Autodesk Fusion 360 part; units mm, degrees
(part 3 of 3)
  spline S752 degree 3 poles (35.1137, 3.9939) (35.046, 4.0714) (34.9934, 4.0943) (34.9088, 4.0943) knots 0 0 0 0 1 1 1 1
  spline S753 degree 3 poles (37.0883, 3.2718) (37.0935, 3.2826) (37.1011, 3.3047) (37.1069, 3.3369) knots 0 0 0 0 0.456304 0.456304 0.456304 0.456304
  spline S754 degree 3 poles (37.1069, 3.3369) (37.0284, 3.3202) (36.9414, 3.3052) (36.8456, 3.2915) knots 0.585455 0.585455 0.585455 0.585455 0.999639 0.999639 0.999639 0.999639
  spline S755 degree 3 poles (36.8456, 3.2915) (36.7271, 3.2744) (36.6453, 3.2517) (36.629, 3.2446) knots 0 0 0 0 1 1 1 1
  spline S756 degree 3 poles (36.629, 3.2446) (36.6076, 3.2353) (36.6025, 3.2294) (36.5959, 3.2194) knots 0.000036 0.000036 0.000036 0.000036 1 1 1 1
  spline S757 degree 3 poles (36.5959, 3.2194) (36.5878, 3.2068) (36.5856, 3.2004) (36.5856, 3.1825) knots 0.000113 0.000113 0.000113 0.000113 1 1 1 1
  spline S758 degree 3 poles (36.5856, 3.1825) (36.5856, 3.1511) (36.586, 3.1497) (36.6107, 3.1279) knots 0 0 0 0 1 1 1 1
  spline S759 degree 3 poles (36.6107, 3.1279) (36.6249, 3.1155) (36.6616, 3.096) (36.7505, 3.096) knots 0.000045 0.000045 0.000045 0.000045 1 1 1 1
  spline S760 degree 3 poles (36.7505, 3.096) (36.8396, 3.096) (36.9078, 3.1141) (36.968, 3.1479) knots 0 0 0 0 1 1 1 1
  spline S761 degree 3 poles (36.968, 3.1479) (37.0284, 3.1818) (37.0627, 3.2189) (37.0883, 3.2718) knots 0.000007 0.000007 0.000007 0.000007 0.994861 0.994861 0.994861 0.994861
  spline S762 degree 3 poles (37.8884, 11.0482) (37.867, 11.0389) (37.8618, 11.0329) (37.8553, 11.0229) knots 0.000005 0.000005 0.000005 0.000005 1 1 1 1
  spline S763 degree 3 poles (37.8553, 11.0229) (37.8471, 11.0103) (37.845, 11.004) (37.845, 10.986) knots 0 0 0 0 1 1 1 1
  spline S764 degree 3 poles (37.845, 10.986) (37.845, 10.9546) (37.8453, 10.9533) (37.8701, 10.9315) knots 0 0 0 0 1 1 1 1
  spline S765 degree 3 poles (37.8701, 10.9315) (37.8842, 10.919) (37.921, 10.8995) (38.0099, 10.8995) knots 0 0 0 0 1 1 1 1
  spline S766 degree 3 poles (38.0099, 10.8995) (38.099, 10.8995) (38.1672, 10.9177) (38.2274, 10.9515) knots 0 0 0 0 1 1 1 1
  spline S767 degree 3 poles (38.2274, 10.9515) (38.2878, 10.9854) (38.3221, 11.0224) (38.3477, 11.0753) knots 0 0 0 0 0.994864 0.994864 0.994864 0.994864
  spline S768 degree 3 poles (38.3477, 11.0753) (38.3528, 11.0862) (38.3605, 11.1082) (38.3663, 11.1404) knots 0 0 0 0 0.4563 0.4563 0.4563 0.4563
  spline S769 degree 3 poles (38.3663, 11.1404) (38.2878, 11.1238) (38.2008, 11.1087) (38.1049, 11.095) knots 0.585457 0.585457 0.585457 0.585457 0.999641 0.999641 0.999641 0.999641
  spline S770 degree 3 poles (38.1049, 11.095) (37.9865, 11.078) (37.9046, 11.0552) (37.8884, 11.0482) knots 0 0 0 0 1 1 1 1
  spline S771 degree 3 poles (41.9828, 11.4158) (41.9828, 11.6094) (41.9395, 11.7253) (41.8802, 11.7925) knots 0 0 0 0 1 1 1 1
  spline S772 degree 3 poles (41.8802, 11.7925) (41.8109, 11.8711) (41.7511, 11.8979) (41.6507, 11.8979) knots 0 0 0 0 1 1 1 1
  spline S773 degree 3 poles (41.6507, 11.8979) (41.5471, 11.8979) (41.4868, 11.8706) (41.4188, 11.7934) knots 0 0 0 0 1 1 1 1
  spline S774 degree 3 poles (41.4188, 11.7934) (41.3618, 11.7287) (41.317, 11.6084) (41.317, 11.4055) knots 0.000006 0.000006 0.000006 0.000006 1 1 1 1
  spline S775 degree 3 poles (41.317, 11.4055) (41.317, 11.2027) (41.3617, 11.0819) (41.4191, 11.0164) knots 0 0 0 0 1 1 1 1
  spline S776 degree 3 poles (41.4191, 11.0164) (41.4873, 10.9387) (41.5474, 10.9115) (41.6507, 10.9115) knots 0.000005 0.000005 0.000005 0.000005 1 1 1 1
  spline S777 degree 3 poles (41.6507, 10.9115) (41.7523, 10.9115) (41.8118, 10.9384) (41.8803, 11.0169) knots 0 0 0 0 1 1 1 1
  spline S778 degree 3 poles (41.8803, 11.0169) (41.937, 11.0819) (41.9828, 11.2065) (41.9828, 11.4158) knots 0.000006 0.000006 0.000006 0.000006 1 1 1 1
  spline S779 degree 3 poles (39.2584, 7.9101) (39.1924, 7.9899) (39.1461, 8.0098) (39.0723, 8.0098) knots 0.000011 0.000011 0.000011 0.000011 1 1 1 1
  spline S780 degree 3 poles (39.0723, 8.0098) (39.0039, 8.0098) (38.9533, 7.9887) (38.8797, 7.8993) knots 0 0 0 0 1 1 1 1
  spline S781 degree 3 poles (38.8797, 7.8993) (38.8187, 7.8253) (38.7744, 7.6978) (38.7744, 7.4935) knots 0.00001 0.00001 0.00001 0.00001 1 1 1 1
  spline S782 degree 3 poles (38.7744, 7.4935) (38.7744, 7.2875) (38.8186, 7.165) (38.8685, 7.1061) knots 0 0 0 0 1 1 1 1
  spline S783 degree 3 poles (38.8685, 7.1061) (38.9327, 7.0303) (38.9799, 7.0097) (39.0587, 7.0097) knots 0.000011 0.000011 0.000011 0.000011 1 1 1 1
  spline S784 degree 3 poles (39.0587, 7.0097) (39.1387, 7.0097) (39.1886, 7.0315) (39.2561, 7.1116) knots 0 0 0 0 1 1 1 1
  spline S785 degree 3 poles (39.2561, 7.1116) (39.3089, 7.1743) (39.3549, 7.3037) (39.3549, 7.5191) knots 0 0 0 0 1 1 1 1
  spline S786 degree 3 poles (39.3549, 7.5191) (39.3549, 7.7225) (39.3114, 7.846) (39.2584, 7.9101) knots 0 0 0 0 1 1 1 1
  spline S787 degree 3 poles (43.6795, 7.9136) (43.6679, 7.9022) (43.6578, 7.8905) (43.6483, 7.8777) knots 0 0 0 0 0.197473 0.197473 0.197473 0.197473
  line L387 (43.6483, 7.8777) -> (44.1325, 7.8777)
  spline S788 degree 3 poles (44.1325, 7.8777) (44.1293, 7.8826) (44.1262, 7.8868) (44.1231, 7.8906) knots 0.866058 0.866058 0.866058 0.866058 0.982774 0.982774 0.982774 0.982774
  spline S789 degree 3 poles (44.1231, 7.8906) (44.1225, 7.8914) (44.1218, 7.8922) (44.1211, 7.893) (44.0566, 7.9711) (44.0001, 7.9978) (43.895, 7.9978) knots -0.006904 -0.006904 -0.006904 -0.006904 0 0 0 1 1 1 1
  spline S790 degree 3 poles (43.895, 7.9978) (43.7986, 7.9978) (43.7407, 7.9737) (43.6795, 7.9136) knots 0 0 0 0 1 1 1 1
  spline S791 degree 3 poles (40.3914, 4.0943) (40.2878, 4.0943) (40.2275, 4.0671) (40.1594, 3.9899) knots 0 0 0 0 1 1 1 1
  spline S792 degree 3 poles (40.1594, 3.9899) (40.1024, 3.9252) (40.0576, 3.8048) (40.0576, 3.602) knots 0.000005 0.000005 0.000005 0.000005 1 1 1 1
  spline S793 degree 3 poles (40.0576, 3.602) (40.0576, 3.3991) (40.1024, 3.2783) (40.1598, 3.2129) knots 0 0 0 0 1 1 1 1
  spline S794 degree 3 poles (40.1598, 3.2129) (40.2279, 3.1352) (40.288, 3.1079) (40.3914, 3.1079) knots 0.000003 0.000003 0.000003 0.000003 1 1 1 1
  spline S795 degree 3 poles (40.3914, 3.1079) (40.493, 3.1079) (40.5525, 3.1349) (40.621, 3.2133) knots 0 0 0 0 1 1 1 1
  spline S796 degree 3 poles (40.621, 3.2133) (40.6777, 3.2783) (40.7234, 3.403) (40.7234, 3.6122) knots 0.000006 0.000006 0.000006 0.000006 1 1 1 1
  spline S797 degree 3 poles (40.7234, 3.6122) (40.7234, 3.8059) (40.6801, 3.9217) (40.6208, 3.989) knots 0 0 0 0 1 1 1 1
  spline S798 degree 3 poles (40.6208, 3.989) (40.5515, 4.0675) (40.4917, 4.0943) (40.3914, 4.0943) knots 0 0 0 0 1 1 1 1
  spline S799 degree 3 poles (45.0503, 4.0943) (44.9467, 4.0943) (44.8864, 4.0671) (44.8184, 3.9899) knots 0 0 0 0 1 1 1 1
  spline S800 degree 3 poles (44.8184, 3.9899) (44.7613, 3.9252) (44.7165, 3.8048) (44.7165, 3.602) knots 0.000005 0.000005 0.000005 0.000005 1 1 1 1
  spline S801 degree 3 poles (44.7165, 3.602) (44.7165, 3.3991) (44.7613, 3.2783) (44.8187, 3.2129) knots 0 0 0 0 1 1 1 1
  spline S802 degree 3 poles (44.8187, 3.2129) (44.8868, 3.1352) (44.947, 3.1079) (45.0503, 3.1079) knots 0.000003 0.000003 0.000003 0.000003 1 1 1 1
  spline S803 degree 3 poles (45.0503, 3.1079) (45.1519, 3.1079) (45.2114, 3.1349) (45.2799, 3.2133) knots 0 0 0 0 1 1 1 1
  spline S804 degree 3 poles (45.2799, 3.2133) (45.3366, 3.2783) (45.3824, 3.403) (45.3824, 3.6122) knots 0.000006 0.000006 0.000006 0.000006 1 1 1 1
  spline S805 degree 3 poles (45.3824, 3.6122) (45.3824, 3.8059) (45.339, 3.9217) (45.2797, 3.989) knots 0 0 0 0 1 1 1 1
  spline S806 degree 3 poles (45.2797, 3.989) (45.2105, 4.0675) (45.1506, 4.0943) (45.0503, 4.0943) knots 0 0 0 0 1 1 1 1
  dimension "d2" = 60
  dimension "d3" = 1
  dimension "d5" = 35
  dimension "d7" = 5
  dimension "d18" = -0.2
  dimension "d19" = -0.2
  dimension "d20" = -0.2
  dimension "d21" = -0.2
  dimension "d22" = -0.2
  dimension "d23" = -0.2
  dimension "d24" = -0.2
  dimension "d25" = -0.2
  dimension "d26" = -0.2
  dimension "d27" = -0.2
  dimension "d28" = -0.2
  dimension "d29" = -0.2
  dimension "d30" = -0.2
  dimension "d31" = -0.2
  dimension "d32" = -0.2
  dimension "d33" = -0.2
  dimension "d34" = -0.2
  dimension "d35" = -0.2
  dimension "d36" = -0.2
  dimension "d37" = -0.2
  dimension "d38" = -0.2
  dimension "d39" = -0.2
  dimension "d40" = -0.2
  constraint parallel L0 L2
  constraint coincident L0 L3.end
  constraint perpendicular L1 L3
  constraint perpendicular L6 L7
  constraint parallel L5 L8
  constraint perpendicular L8 L9
  constraint coincident L9 L10.start
  constraint perpendicular L9 L10
  constraint coincident L9 L11.end
  constraint coincident L7 L11.end
  constraint coincident L6 L12.end
  constraint coincident L12 L13.start
  constraint vertical L13
  constraint coincident L6 L14.end
  constraint parallel L12 L14
  constraint coincident L5 L15.start
  constraint perpendicular L5 L15
  constraint perpendicular L15 L16
  constraint perpendicular L16 L17
  constraint horizontal L18
  constraint perpendicular L16 L19
  constraint parallel L18 L20
  constraint coincident L5 L21.end
  constraint perpendicular L5 L21
  constraint parallel L19 L22
  constraint coincident L5 L23.end
  constraint vertical L23
  constraint perpendicular L5 L24
  constraint perpendicular L5 L25
  constraint coincident L21 L27.end
  constraint parallel L20 L27
  constraint coincident L21 L28.start
  constraint horizontal L28
  constraint horizontal L30
  constraint parallel L30 L32
  constraint parallel L32 L34
  constraint coincident L5 L36.end
  constraint parallel L34 L36
  constraint coincident L37 L39.end
  constraint coincident L5 L42.start
  constraint coincident L9.end L12
  constraint horizontal L43
  constraint coincident L0.start L43
  constraint perpendicular L16 L45
  constraint coincident L5 L46.end
  constraint vertical L46
  constraint coincident L44 L47.start
  constraint horizontal L48
  constraint vertical L49
  constraint horizontal L50
  constraint vertical L51
  constraint perpendicular L43 L54
  measures "d2" distance of L48.start L48.end
  measures "d5" distance of L48 L50
  measures "d7" diameter of A0
extrude "Estrusione2" add sketch "Schizzo1" along normal blind 2 contours L0 L4 L5 L42 | L43 L52 L53 L54 | L0 L1 L2 L3 | L5 L6 L42 | L5 L37 L39 | L32 L35 L36 L37 L38 L41 | L6 L12 L13 L14 | L5 L15 L16 L45 L46 | L5 L44 L47 | L21 L28 L31 L37 L38 L39 L40 | L19 L20 L21 L22 L44 | L6 L7 L9 L12 | L17 L18 L22 L44 L45 L46 L47 | L33 L34 L41 | L7 L8 L9 | L21 L26 L27 | L29 L30 L40 | L7 L9 L12 | L9 L10 L11 | L48 L49 L50 L51 | L55 L56 L57 S0 S1 L58 L59 L60 L61 L62 L63 L64 L65 L66 L67 | S2 S3 S4 S5 S6 S7 S8 S9 S10 | S11 S12 S13 S14 S15 S16 S17 S18 | L68 L69 L70 S19 S20 S21 S22 S23 L71 L72 L73 S24 S25 S26 S27 S28 L74 L75 | L76 S29 S30 S31 S32 L77 L78 L79 L80 L81 L82 L83 L84 L85 L86 L87 S33 S34 S35 S36 | L88 S37 S38 S39 S40 S41 S42 S43 S44 S45 L89 S46 S47 S48 S49 | L90 S50 S51 S52 S53 | L91 L92 S54 S55 S56 S57 S58 S59 S60 S61 S62 L93 | L94 S63 S64 S65 S66 S67 S68 S69 L95 L96 | L97 S70 S71 S72 S73 S74 S75 S76 S77 S78 L98 S79 S80 S81 S82 | L99 S83 S84 S85 S86 | L100 L101 L102 L103 | L104 L105 L106 S87 S88 S89 S90 S91 S92 S93 S94 S95 S96 S97 L107 S98 S99 S100 S101 S102 S103 S104 S105 S106 S107 S108 S109 L108 L109 | S110 S111 S112 S113 S114 S115 S116 S117 S118 S119 S120 S121 S122 S123 L110 S124 S125 S126 S127 S128 S129 S130 L111 S131 S132 L112 S133 | S134 S135 S136 S137 S138 S139 S140 S141 S142 L113 | L114 L115 L116 L117 | L118 L119 L120 L121 | S143 S144 S145 S146 S147 S148 S149 S150 S151 | S152 S153 S154 S155 S156 S157 S158 S159 | L122 S160 S161 S162 S163 S164 S165 S166 S167 S168 S169 S170 S171 S172 S173 S174 S175 S176 S177 L123 S178 S179 S180 S181 S182 S183 S184 S185 S186 S187 S188 S189 S190 S191 S192 | S193 S194 S195 S196 S197 S198 S199 S200 S201 | S202 S203 S204 S205 S206 S207 S208 S209 | L124 L125 L126 L127 L128 S210 S211 S212 S213 L129 S214 S215 S216 L130 L131 L132 L133 L134 L135 | L136 S217 S218 S219 S220 L137 L138 L139 L140 L141 L142 L143 L144 L145 L146 L147 S221 S222 S223 S224 | L148 L149 L150 L151 S225 L152 L153 L154 L155 L156 L157 L158 L159 L160 L161 L162 L163 L164 | S226 S227 S228 S229 S230 S231 S232 S233 S234 S235 S236 S237 S238 S239 L165 S240 S241 S242 S243 S244 S245 S246 L166 S247 S248 L167 S249 | S250 S251 S252 S253 S254 S255 S256 S257 S258 L168 | L169 L170 L171 S259 S260 S261 L172 S262 S263 S264 S265 L173 L174 | L175 S266 S267 S268 S269 S270 S271 S272 S273 S274 L176 S275 S276 S277 S278 | L177 S279 S280 S281 S282 | L178 L179 S283 S284 S285 S286 S287 S288 S289 S290 S291 L180 | L181 S292 S293 S294 S295 S296 S297 S298 L182 L183 | L184 S299 S300 S301 S302 S303 S304 S305 S306 S307 L185 S308 S309 S310 S311 | L186 S312 S313 S314 S315 | L187 L188 L189 S316 S317 L190 L191 L192 L193 | L194 S318 S319 S320 S321 S322 S323 S324 S325 S326 L195 S327 S328 S329 S330 | L196 S331 S332 S333 S334 | L197 L198 L199 L200 | S335 S336 S337 S338 S339 S340 S341 S342 S343 | S344 S345 S346 S347 S348 S349 S350 S351 | L201 L202 L203 S352 S353 S354 S355 S356 S357 S358 S359 S360 S361 L204 L205 | S362 S363 S364 S365 S366 S367 S368 S369 | L206 L207 L208 S370 S371 S372 S373 S374 S375 S376 L209 L210 L211 S377 S378 S379 S380 S381 L212 L213 L214 S382 S383 S384 S385 S386 L215 L216 | L217 S387 S388 S389 S390 S391 S392 S393 S394 S395 L218 S396 S397 S398 S399 | L219 S400 S401 S402 S403 | L220 L221 L222 S404 S405 S406 S407 S408 L223 L224 L225 S409 S410 S411 S412 S413 L226 L227 | L228 S414 S415 S416 S417 L229 L230 L231 L232 L233 L234 L235 L236 L237 L238 L239 S418 S419 S420 S421 | L240 L241 L242 L243 S422 L244 L245 L246 L247 L248 L249 L250 L251 L252 L253 L254 L255 L256 | L257 L258 L259 L260 S423 L261 L262 L263 L264 L265 L266 L267 L268 L269 L270 L271 L272 L273 | L274 L275 L276 L277 S424 L278 L279 L280 L281 L282 L283 L284 L285 L286 L287 L288 L289 L290 | L291 L292 L293 L294 | L295 L296 L297 S425 S426 S427 S428 S429 S430 S431 L298 L299 L300 S432 S433 S434 S435 S436 L301 L302 L303 S437 S438 S439 S440 S441 L304 L305 | S442 S443 S444 S445 S446 S447 S448 S449 S450 | S451 S452 S453 S454 S455 S456 S457 S458 | L306 L307 L308 S459 S460 S461 S462 S463 L309 L310 L311 S464 S465 S466 S467 S468 L312 L313 | L314 S469 S470 S471 S472 L315 L316 L317 L318 L319 L320 L321 L322 L323 L324 L325 S473 S474 S475 S476 | L326 S477 S478 S479 S480 S481 S482 S483 S484 S485 L327 S486 S487 S488 S489 | L328 S490 S491 S492 S493 | L329 S494 S495 S496 S497 S498 S499 S500 S501 S502 L330 L331 L332 L333 | S503 S504 S505 S506 S507 S508 S509 S510 | L334 S511 S512 S513 S514 S515 S516 S517 S518 S519 L335 S520 S521 S522 S523 | L336 S524 S525 S526 S527 | L337 L338 L339 L340 | L341 S528 S529 S530 S531 S532 S533 S534 S535 S536 S537 S538 S539 L342 L343 L344 S540 S541 S542 S543 S544 | S545 S546 S547 S548 S549 S550 S551 S552 | S553 S554 S555 S556 S557 S558 S559 S560 S561 S562 S563 S564 S565 S566 L345 S567 S568 S569 S570 S571 S572 S573 L346 S574 S575 L347 S576 | S577 S578 S579 S580 S581 S582 S583 S584 S585 L348 | L349 L350 L351 L352 | L353 L354 L355 L356 | S586 S587 S588 S589 S590 S591 S592 S593 S594 | S595 S596 S597 S598 S599 S600 S601 S602 | L357 L358 L359 L360 | L361 S603 S604 S605 S606 S607 S608 S609 S610 S611 L362 S612 S613 S614 S615 S616 S617 S618 S619 | S620 S621 S622 S623 S624 S625 S626 S627 S628 | S629 S630 S631 S632 S633 S634 S635 S636 | L363 L364 L365 S637 S638 S639 S640 S641 S642 S643 L366 L367 L368 S644 S645 S646 S647 S648 L369 L370 L371 S649 S650 S651 S652 S653 L372 L373 | A0 | S654 S655 S656 S657 S658 S659 S660 S661 | L374 S662 S663 S664 S665 | L375 S666 S667 S668 S669 S670 S671 S672 L376 L377 | S673 L378 S674 S675 S676 | S677 S678 S679 S680 S681 S682 S683 S684 | S685 S686 S687 S688 S689 S690 S691 S692 S693 | L379 S694 S695 S696 S697 | L380 L381 S698 S699 S700 S701 S702 S703 S704 L382 | S705 S706 S707 L383 S708 | S709 S710 S711 L384 S712 | S713 S714 S715 S716 S717 S718 S719 S720 | S721 S722 S723 S724 S725 S726 S727 S728 | S729 L385 S730 S731 S732 | S733 S734 S735 S736 S737 S738 S739 S740 | S741 L386 S742 S743 S744 | S745 S746 S747 S748 S749 S750 S751 S752 | S753 S754 S755 S756 S757 S758 S759 S760 S761 | S762 S763 S764 S765 S766 S767 S768 S769 S770 | S771 S772 S773 S774 S775 S776 S777 S778 | S779 S780 S781 S782 S783 S784 S785 S786 | S787 L387 S788 S789 S790 | S791 S792 S793 S794 S795 S796 S797 S798 | S799 S800 S801 S802 S803 S804 S805 S806 picked at (32.5784, 24.2635) picked at (29.7633, 19.2235) picked at (33.4667, 23.0128) picked at (32.8761, 26.4165) picked at (28.2244, 24.0953) picked at (26.1986, 24.8309) picked at (36.488, 28.9145) picked at (30.7392, 28.8709) picked at (29.0404, 24.8074) picked at (24.6839, 27.2601) picked at (26.287, 28.4268) picked at (36.1096, 29.9049) picked at (27.414, 28.4795) picked at (21.6638, 25.7314) picked at (35.0097, 31.6222) picked at (21.2262, 30.3118) picked at (21.0939, 27.9286) picked at (37.5639, 30.9019) picked at (36.6212, 31.7784) picked at (46.8168, 26.1128) picked at (20.1256, 12.0308) picked at (22.1992, 11.3251) picked at (21.0011, 11.2982) picked at (22.7711, 11.4334) picked at (24.871, 11.372) picked at (26.5894, 11.4112) picked at (26.24, 11.6461) picked at (28.6437, 12.0683) picked at (28.9309, 12.0017) picked at (32.0242, 11.4112) picked at (31.6748, 11.6461) picked at (33.0542, 12.1667) picked at (36.8651, 11.368) picked at (38.7811, 11.0053) picked at (38.2506, 11.1875) picked at (39.4594, 12.1667) picked at (40.2353, 12.1667) picked at (42.3885, 11.3251) picked at (41.1904, 11.2982) picked at (13.7913, 7.9143) picked at (16.4744, 7.4233) picked at (15.2763, 7.3964) picked at (17.1191, 7.6464) picked at (18.1742, 7.4702) picked at (19.0513, 7.4571) picked at (22.7665, 7.1035) picked at (22.236, 7.2857) picked at (23.4482, 7.518) picked at (25.5201, 7.5094) picked at (25.1707, 7.7444) picked at (27.5745, 8.1666) picked at (27.8617, 7.5966) picked at (30.955, 7.5094) picked at (30.6056, 7.7444) picked at (32.1709, 7.4441) picked at (34.6436, 7.5094) picked at (34.2942, 7.7444) picked at (35.6736, 8.2649) picked at (37.8267, 7.4233) picked at (36.6287, 7.3964) picked at (38.3933, 7.2045) picked at (38.6489, 7.3746) picked at (40.3411, 7.5151) picked at (44.1559, 7.5094) picked at (43.8065, 7.7444) picked at (45.1927, 7.5316) picked at (47.2925, 7.4702) picked at (11.6749, 3.5554) picked at (14.1971, 3.5554) picked at (16.7192, 3.5554) picked at (19.0857, 2.9295) picked at (19.9548, 3.6133) picked at (24.2345, 3.5215) picked at (23.0364, 3.4946) picked at (24.8064, 3.6298) picked at (26.9063, 3.5684) picked at (28.6247, 3.6077) picked at (28.2753, 3.8426) picked at (30.9214, 3.891) picked at (30.6645, 3.702) picked at (32.5094, 3.6077) picked at (32.16, 3.8426) picked at (33.5394, 4.3631) picked at (35.6028, 3.6912) picked at (34.4922, 3.5133) picked at (37.5218, 3.2018) picked at (36.9913, 3.384) picked at (38.2, 4.3631) picked at (38.976, 4.3631) picked at (41.1291, 3.5215) picked at (39.931, 3.4946) picked at (41.8022, 2.9295) picked at (42.691, 3.4971) picked at (45.788, 3.5215) picked at (44.5899, 3.4946) picked at (46.36, 3.6133) picked at (4.7162, 31.8393) picked at (21.466, 11.016) picked at (26.3254, 11.8195) picked at (29.6156, 11.7563) picked at (31.7603, 11.8195) picked at (15.7412, 7.1142) picked at (22.0347, 7.1206) picked at (25.2562, 7.9177) picked at (28.5463, 7.8545) picked at (30.691, 7.9177) picked at (34.3796, 7.9177) picked at (37.0935, 7.1142) picked at (23.5013, 3.2124) picked at (28.3607, 4.016) picked at (30.3445, 3.6715) picked at (32.2454, 4.016) picked at (34.8186, 3.5484) picked at (36.79, 3.2189) picked at (38.0494, 11.0224) picked at (41.6553, 11.016) picked at (38.9706, 7.4191) picked at (43.8919, 7.9177) picked at (40.3959, 3.2124) picked at (45.0548, 3.2124)
extrude "Estrusione3" cut 1 faces at (20, 23.3176, 2) along direction (0, 0, -1) blind 2
extrude "Estrusione4" add sketch "Schizzo1" against normal blind 2 contours L0 L4 L5 L42 | L43 L52 L53 L54 | L0 L1 L2 L3 | L5 L6 L42 | L5 L37 L39 | L32 L35 L36 L37 L38 L41 | L6 L12 L13 L14 | L5 L15 L16 L45 L46 | L5 L44 L47 | L21 L28 L31 L37 L38 L39 L40 | L19 L20 L21 L22 L44 | L6 L7 L9 L12 | L17 L18 L22 L44 L45 L46 L47 | L33 L34 L41 | L7 L8 L9 | L21 L26 L27 | L29 L30 L40 | L7 L9 L12 | L9 L10 L11 | L48 L49 L50 L51 | L55 L56 L57 S0 S1 L58 L59 L60 L61 L62 L63 L64 L65 L66 L67 | S2 S3 S4 S5 S6 S7 S8 S9 S10 | S11 S12 S13 S14 S15 S16 S17 S18 | L68 L69 L70 S19 S20 S21 S22 S23 L71 L72 L73 S24 S25 S26 S27 S28 L74 L75 | L76 S29 S30 S31 S32 L77 L78 L79 L80 L81 L82 L83 L84 L85 L86 L87 S33 S34 S35 S36 | L88 S37 S38 S39 S40 S41 S42 S43 S44 S45 L89 S46 S47 S48 S49 | L90 S50 S51 S52 S53 | L91 L92 S54 S55 S56 S57 S58 S59 S60 S61 S62 L93 | L94 S63 S64 S65 S66 S67 S68 S69 L95 L96 | L97 S70 S71 S72 S73 S74 S75 S76 S77 S78 L98 S79 S80 S81 S82 | L99 S83 S84 S85 S86 | L100 L101 L102 L103 | L104 L105 L106 S87 S88 S89 S90 S91 S92 S93 S94 S95 S96 S97 L107 S98 S99 S100 S101 S102 S103 S104 S105 S106 S107 S108 S109 L108 L109 | S110 S111 S112 S113 S114 S115 S116 S117 S118 S119 S120 S121 S122 S123 L110 S124 S125 S126 S127 S128 S129 S130 L111 S131 S132 L112 S133 | S134 S135 S136 S137 S138 S139 S140 S141 S142 L113 | L114 L115 L116 L117 | L118 L119 L120 L121 | S143 S144 S145 S146 S147 S148 S149 S150 S151 | S152 S153 S154 S155 S156 S157 S158 S159 | L122 S160 S161 S162 S163 S164 S165 S166 S167 S168 S169 S170 S171 S172 S173 S174 S175 S176 S177 L123 S178 S179 S180 S181 S182 S183 S184 S185 S186 S187 S188 S189 S190 S191 S192 | S193 S194 S195 S196 S197 S198 S199 S200 S201 | S202 S203 S204 S205 S206 S207 S208 S209 | L124 L125 L126 L127 L128 S210 S211 S212 S213 L129 S214 S215 S216 L130 L131 L132 L133 L134 L135 | L136 S217 S218 S219 S220 L137 L138 L139 L140 L141 L142 L143 L144 L145 L146 L147 S221 S222 S223 S224 | L148 L149 L150 L151 S225 L152 L153 L154 L155 L156 L157 L158 L159 L160 L161 L162 L163 L164 | S226 S227 S228 S229 S230 S231 S232 S233 S234 S235 S236 S237 S238 S239 L165 S240 S241 S242 S243 S244 S245 S246 L166 S247 S248 L167 S249 | S250 S251 S252 S253 S254 S255 S256 S257 S258 L168 | L169 L170 L171 S259 S260 S261 L172 S262 S263 S264 S265 L173 L174 | L175 S266 S267 S268 S269 S270 S271 S272 S273 S274 L176 S275 S276 S277 S278 | L177 S279 S280 S281 S282 | L178 L179 S283 S284 S285 S286 S287 S288 S289 S290 S291 L180 | L181 S292 S293 S294 S295 S296 S297 S298 L182 L183 | L184 S299 S300 S301 S302 S303 S304 S305 S306 S307 L185 S308 S309 S310 S311 | L186 S312 S313 S314 S315 | L187 L188 L189 S316 S317 L190 L191 L192 L193 | L194 S318 S319 S320 S321 S322 S323 S324 S325 S326 L195 S327 S328 S329 S330 | L196 S331 S332 S333 S334 | L197 L198 L199 L200 | S335 S336 S337 S338 S339 S340 S341 S342 S343 | S344 S345 S346 S347 S348 S349 S350 S351 | L201 L202 L203 S352 S353 S354 S355 S356 S357 S358 S359 S360 S361 L204 L205 | S362 S363 S364 S365 S366 S367 S368 S369 | L206 L207 L208 S370 S371 S372 S373 S374 S375 S376 L209 L210 L211 S377 S378 S379 S380 S381 L212 L213 L214 S382 S383 S384 S385 S386 L215 L216 | L217 S387 S388 S389 S390 S391 S392 S393 S394 S395 L218 S396 S397 S398 S399 | L219 S400 S401 S402 S403 | L220 L221 L222 S404 S405 S406 S407 S408 L223 L224 L225 S409 S410 S411 S412 S413 L226 L227 | L228 S414 S415 S416 S417 L229 L230 L231 L232 L233 L234 L235 L236 L237 L238 L239 S418 S419 S420 S421 | L240 L241 L242 L243 S422 L244 L245 L246 L247 L248 L249 L250 L251 L252 L253 L254 L255 L256 | L257 L258 L259 L260 S423 L261 L262 L263 L264 L265 L266 L267 L268 L269 L270 L271 L272 L273 | L274 L275 L276 L277 S424 L278 L279 L280 L281 L282 L283 L284 L285 L286 L287 L288 L289 L290 | L291 L292 L293 L294 | L295 L296 L297 S425 S426 S427 S428 S429 S430 S431 L298 L299 L300 S432 S433 S434 S435 S436 L301 L302 L303 S437 S438 S439 S440 S441 L304 L305 | S442 S443 S444 S445 S446 S447 S448 S449 S450 | S451 S452 S453 S454 S455 S456 S457 S458 | L306 L307 L308 S459 S460 S461 S462 S463 L309 L310 L311 S464 S465 S466 S467 S468 L312 L313 | L314 S469 S470 S471 S472 L315 L316 L317 L318 L319 L320 L321 L322 L323 L324 L325 S473 S474 S475 S476 | L326 S477 S478 S479 S480 S481 S482 S483 S484 S485 L327 S486 S487 S488 S489 | L328 S490 S491 S492 S493 | L329 S494 S495 S496 S497 S498 S499 S500 S501 S502 L330 L331 L332 L333 | S503 S504 S505 S506 S507 S508 S509 S510 | L334 S511 S512 S513 S514 S515 S516 S517 S518 S519 L335 S520 S521 S522 S523 | L336 S524 S525 S526 S527 | L337 L338 L339 L340 | L341 S528 S529 S530 S531 S532 S533 S534 S535 S536 S537 S538 S539 L342 L343 L344 S540 S541 S542 S543 S544 | S545 S546 S547 S548 S549 S550 S551 S552 | S553 S554 S555 S556 S557 S558 S559 S560 S561 S562 S563 S564 S565 S566 L345 S567 S568 S569 S570 S571 S572 S573 L346 S574 S575 L347 S576 | S577 S578 S579 S580 S581 S582 S583 S584 S585 L348 | L349 L350 L351 L352 | L353 L354 L355 L356 | S586 S587 S588 S589 S590 S591 S592 S593 S594 | S595 S596 S597 S598 S599 S600 S601 S602 | L357 L358 L359 L360 | L361 S603 S604 S605 S606 S607 S608 S609 S610 S611 L362 S612 S613 S614 S615 S616 S617 S618 S619 | S620 S621 S622 S623 S624 S625 S626 S627 S628 | S629 S630 S631 S632 S633 S634 S635 S636 | L363 L364 L365 S637 S638 S639 S640 S641 S642 S643 L366 L367 L368 S644 S645 S646 S647 S648 L369 L370 L371 S649 S650 S651 S652 S653 L372 L373 | A0 | S654 S655 S656 S657 S658 S659 S660 S661 | L374 S662 S663 S664 S665 | L375 S666 S667 S668 S669 S670 S671 S672 L376 L377 | S673 L378 S674 S675 S676 | S677 S678 S679 S680 S681 S682 S683 S684 | S685 S686 S687 S688 S689 S690 S691 S692 S693 | L379 S694 S695 S696 S697 | L380 L381 S698 S699 S700 S701 S702 S703 S704 L382 | S705 S706 S707 L383 S708 | S709 S710 S711 L384 S712 | S713 S714 S715 S716 S717 S718 S719 S720 | S721 S722 S723 S724 S725 S726 S727 S728 | S729 L385 S730 S731 S732 | S733 S734 S735 S736 S737 S738 S739 S740 | S741 L386 S742 S743 S744 | S745 S746 S747 S748 S749 S750 S751 S752 | S753 S754 S755 S756 S757 S758 S759 S760 S761 | S762 S763 S764 S765 S766 S767 S768 S769 S770 | S771 S772 S773 S774 S775 S776 S777 S778 | S779 S780 S781 S782 S783 S784 S785 S786 | S787 L387 S788 S789 S790 | S791 S792 S793 S794 S795 S796 S797 S798 | S799 S800 S801 S802 S803 S804 S805 S806 picked at (32.5784, 24.2635) picked at (29.7633, 19.2235) picked at (33.4667, 23.0128) picked at (32.8761, 26.4165) picked at (28.2244, 24.0953) picked at (26.1986, 24.8309) picked at (36.488, 28.9145) picked at (30.7392, 28.8709) picked at (29.0404, 24.8074) picked at (24.6839, 27.2601) picked at (26.287, 28.4268) picked at (36.1096, 29.9049) picked at (27.414, 28.4795) picked at (21.6638, 25.7314) picked at (35.0097, 31.6222) picked at (21.2262, 30.3118) picked at (21.0939, 27.9286) picked at (37.5639, 30.9019) picked at (36.6212, 31.7784) picked at (46.8168, 26.1128) picked at (20.1256, 12.0308) picked at (22.1992, 11.3251) picked at (21.0011, 11.2982) picked at (22.7711, 11.4334) picked at (24.871, 11.372) picked at (26.5894, 11.4112) picked at (26.24, 11.6461) picked at (28.6437, 12.0683) picked at (28.9309, 12.0017) picked at (32.0242, 11.4112) picked at (31.6748, 11.6461) picked at (33.0542, 12.1667) picked at (36.8651, 11.368) picked at (38.7811, 11.0053) picked at (38.2506, 11.1875) picked at (39.4594, 12.1667) picked at (40.2353, 12.1667) picked at (42.3885, 11.3251) picked at (41.1904, 11.2982) picked at (13.7913, 7.9143) picked at (16.4744, 7.4233) picked at (15.2763, 7.3964) picked at (17.1191, 7.6464) picked at (18.1742, 7.4702) picked at (19.0513, 7.4571) picked at (22.7665, 7.1035) picked at (22.236, 7.2857) picked at (23.4482, 7.518) picked at (25.5201, 7.5094) picked at (25.1707, 7.7444) picked at (27.5745, 8.1666) picked at (27.8617, 7.5966) picked at (30.955, 7.5094) picked at (30.6056, 7.7444) picked at (32.1709, 7.4441) picked at (34.6436, 7.5094) picked at (34.2942, 7.7444) picked at (35.6736, 8.2649) picked at (37.8267, 7.4233) picked at (36.6287, 7.3964) picked at (38.3933, 7.2045) picked at (38.6489, 7.3746) picked at (40.3411, 7.5151) picked at (44.1559, 7.5094) picked at (43.8065, 7.7444) picked at (45.1927, 7.5316) picked at (47.2925, 7.4702) picked at (11.6749, 3.5554) picked at (14.1971, 3.5554) picked at (16.7192, 3.5554) picked at (19.0857, 2.9295) picked at (19.9548, 3.6133) picked at (24.2345, 3.5215) picked at (23.0364, 3.4946) picked at (24.8064, 3.6298) picked at (26.9063, 3.5684) picked at (28.6247, 3.6077) picked at (28.2753, 3.8426) picked at (30.9214, 3.891) picked at (30.6645, 3.702) picked at (32.5094, 3.6077) picked at (32.16, 3.8426) picked at (33.5394, 4.3631) picked at (35.6028, 3.6912) picked at (34.4922, 3.5133) picked at (37.5218, 3.2018) picked at (36.9913, 3.384) picked at (38.2, 4.3631) picked at (38.976, 4.3631) picked at (41.1291, 3.5215) picked at (39.931, 3.4946) picked at (41.8022, 2.9295) picked at (42.691, 3.4971) picked at (45.788, 3.5215) picked at (44.5899, 3.4946) picked at (46.36, 3.6133) picked at (4.7162, 31.8393) picked at (21.466, 11.016) picked at (26.3254, 11.8195) picked at (29.6156, 11.7563) picked at (31.7603, 11.8195) picked at (15.7412, 7.1142) picked at (22.0347, 7.1206) picked at (25.2562, 7.9177) picked at (28.5463, 7.8545) picked at (30.691, 7.9177) picked at (34.3796, 7.9177) picked at (37.0935, 7.1142) picked at (23.5013, 3.2124) picked at (28.3607, 4.016) picked at (30.3445, 3.6715) picked at (32.2454, 4.016) picked at (34.8186, 3.5484) picked at (36.79, 3.2189) picked at (38.0494, 11.0224) picked at (41.6553, 11.016) picked at (38.9706, 7.4191) picked at (43.8919, 7.9177) picked at (40.3959, 3.2124) picked at (45.0548, 3.2124)
extrude "Estrusione5" cut sketch "Schizzo1" against normal blind 2 contours A0 picked at (4.7162, 31.8393)
extrude "Estrusione6" add sketch "Schizzo1" along normal blind 4 contours S654 S655 S656 S657 S658 S659 S660 S661 picked at (21.466, 11.016)
extrude "Estrusione7" add sketch "Schizzo1" along normal blind 4 contours L374 S663 S664 | S662 picked at (26.3377, 11.8315) picked at (26.5638, 11.7827)
extrude "Estrusione8" add sketch "Schizzo1" along normal blind 4 contours L375 S666 S667 S668 S669 S670 S671 S672 L376 L377 picked at (29.6156, 11.7563)
extrude "Estrusione9" add sketch "Schizzo1" along normal blind 4 contours S673 L378 S674 S675 S676 picked at (31.7603, 11.8195)
extrude "Estrusione10" add sketch "Schizzo1" along normal blind 4 contours S685 S686 S687 S688 S689 S690 S691 S692 S693 picked at (22.0347, 7.1206)
extrude "Estrusione11" add sketch "Schizzo1" along normal blind 4 contours L379 S695 S696 | S694 picked at (25.2684, 7.9297) picked at (25.4945, 7.881)
extrude "Estrusione12" add sketch "Schizzo1" along normal blind 4 contours L380 L381 S698 S699 S700 S701 S702 S703 S704 L382 picked at (28.5463, 7.8545)
extrude "Estrusione13" add sketch "Schizzo1" along normal blind 4 contours S705 S706 S707 L383 S708 picked at (30.691, 7.9177)
extrude "Estrusione14" add sketch "Schizzo1" along normal blind 4 contours S762 S763 S764 S765 S766 S767 S768 S769 S770 picked at (38.0494, 11.0224)
extrude "Estrusione15" add sketch "Schizzo1" along normal blind 4 contours S771 S772 S773 S774 S775 S776 S777 S778 picked at (41.6553, 11.016)
extrude "Estrusione16" add sketch "Schizzo1" along normal blind 4 contours S709 S710 S711 L384 S712 picked at (34.3796, 7.9177)
extrude "Estrusione17" add sketch "Schizzo1" along normal blind 4 contours S713 S714 S715 S716 S717 S718 S719 S720 picked at (37.0935, 7.1142)
extrude "Estrusione18" add sketch "Schizzo1" along normal blind 4 contours S779 S780 S781 S782 S783 S784 S785 S786 picked at (38.9706, 7.4191)
extrude "Estrusione19" add sketch "Schizzo1" along normal blind 4 contours S787 L387 S788 S789 S790 picked at (43.8919, 7.9177)
extrude "Estrusione20" add sketch "Schizzo1" along normal blind 4 contours S799 S800 S801 S802 S803 S804 S805 S806 picked at (45.0548, 3.2124)
extrude "Estrusione21" add sketch "Schizzo1" along normal blind 4 contours S791 S792 S793 S794 S795 S796 S797 S798 picked at (40.3959, 3.2124)
extrude "Estrusione22" add sketch "Schizzo1" along normal blind 4 contours S753 S754 S755 S756 S757 S758 S759 S760 S761 picked at (36.79, 3.2189)
extrude "Estrusione23" add sketch "Schizzo1" along normal blind 4 contours S745 S746 S747 S748 S749 S750 S751 S752 picked at (34.8186, 3.5484)
extrude "Estrusione24" add sketch "Schizzo1" along normal blind 4 contours S741 L386 S742 S743 S744 picked at (32.2454, 4.016)
extrude "Estrusione25" add sketch "Schizzo1" along normal blind 4 contours S733 S734 S735 S736 S737 S738 S739 S740 picked at (30.3445, 3.6715)
extrude "Estrusione26" add sketch "Schizzo1" along normal blind 4 contours S729 L385 S730 S731 S732 picked at (28.3607, 4.016)
extrude "Estrusione27" add sketch "Schizzo1" along normal blind 4 contours S721 S722 S723 S724 S725 S726 S727 S728 picked at (23.5013, 3.2124)
extrude "Estrusione28" add sketch "Schizzo1" along normal blind 4 contours S677 S678 S679 S680 S681 S682 S683 S684 picked at (15.7412, 7.1142)
